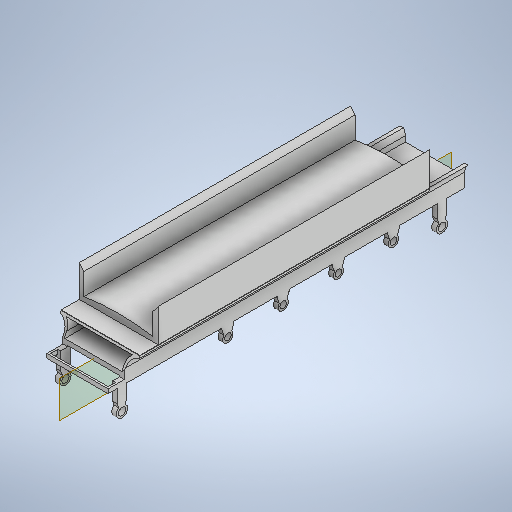
# Autodesk Inventor part: Wheel Holder of Train [Copy]
Saved by Autodesk Inventor 2025.1 (Build 291241020, 241B)
## iProperties
Created: 2022-11-30
Part Number: Wheel Holder of Train [Copy]
Material: Generic
Document SubType Name: Modeling
Designer: mc_vlongo24
Density: 1 g/cm^3
Appearance: Default
Author: mc_vlongo24
Autodesk Inventor part; units mm, degrees
ref_plane "YZ Plane" through (0, 0, 0) normal (1, 0, 0) x (0, 1, 0)
ref_plane "XZ Plane" through (0, 0, 0) normal (0, 1, 0) x (-1, 0, 0)
ref_plane "XY Plane" through (0, 0, 0) normal (0, 0, 1) x (1, 0, 0)
sketch "Sketch1" plane through (0, 0, 0) normal (0, 1, 0) x (-1, 0, 0)
  line L0 (25.5765, 3.2132) -> (-7.4435, 3.2132)
  line L1 (-7.4435, 3.2132) -> (-7.4435, -188.8108)
  line L2 (-7.4435, -188.8108) -> (25.5765, -188.8108)
  line L3 (25.5765, -188.8108) -> (25.5765, 3.2132)
  point P0 (0, 0)
  dimension "d0" = 33.02
  dimension "d1" = 192.024
  constraints: 8 end point, 2 parallel, 1 horizontal, 1 perpendicular
  measures "d0" distance of L2.end L1.end
  measures "d1" distance between parallel lines of L2 L0
extrude "Extrusion1" add sketch "Sketch1" against normal blind 23.8125
sketch "Sketch2" plane through (7.4435, 0, 3.2132) normal (1, 0, 0) x (0, 0, -1)
  line L0 (0, 0) -> (0, -23.8125) projected
  line L1 (192.024, 0) -> (192.024, -23.8125) projected
  line L2 (0, 0) -> (192.024, 0)
  line L3 (192.024, 0) -> (192.024, -20.9629)
  line L4 (192.024, -20.9629) -> (0, -20.9629)
  line L5 (0, -20.9629) -> (0, 0)
  point P0 (3.2132, 0)
  constraints: 8 end point, 2 parallel, 1 horizontal, 1 perpendicular, 1 point on line
extrude "Extrusion2" cut sketch "Sketch2" against normal blind 33.02
sketch "Sketch3" plane through (7.4435, -20.9629, 3.2132) normal (0, 1, 0) x (1, 0, 0)
  line L0 (-32.004, 1.016) -> (-1.016, 1.016)
  line L1 (-1.016, 1.016) -> (-1.016, 191.008)
  line L2 (-1.016, 191.008) -> (-32.004, 191.008)
  line L3 (-32.004, 191.008) -> (-32.004, 1.016)
  line L4 (-33.02, 192.024) -> (0, 192.024) projected
  line L5 (-33.02, 0) -> (-33.02, 192.024) projected
  line L6 (0, 192.024) -> (0, 0) projected
  line L7 (0, 0) -> (-33.02, 0) projected
  point P0 (-7.4435, 3.2132)
  dimension "d6" = 1.016
  dimension "d7" = 1.016
  dimension "d8" = 1.016
  dimension "d9" = 1.016
  constraints: 8 end point, 2 parallel, 1 horizontal, 1 perpendicular
  measures "d6" distance between parallel lines of L4 L2
  measures "d7" distance between parallel lines of L5 L3
  measures "d8" distance between parallel lines of L6 L1
  measures "d9" distance between parallel lines of L7 L0
extrude "Extrusion3" cut sketch "Sketch3" against normal blind 6.0325 contours L3 L2 L1 L0
sketch "Sketch4" plane through (7.4435, -23.8125, 3.2132) normal (1, 0, 0) x (0, 0, -1)
  line L0 (1.016, 2.8496) -> (191.008, 2.8496) projected
  line L1 (4.9428, 2.8496) -> (10.0228, 2.8496)
  line L2 (10.0228, 2.8496) -> (10.0228, -7.1834)
  line L3 (10.0228, -7.1834) -> (4.9428, -7.1834)
  line L4 (4.9428, -7.1834) -> (4.9428, 2.8496)
  circle A0 centre (7.4828, -12.0073) radius 2.032
  circle A1 centre (7.4828, -12.0073) radius 3.048
  line L5 (4.9428, -7.1834) -> (5.7788, -9.4802)
  line L6 (10.0228, -7.1834) -> (9.1869, -9.4802)
  circle A2 centre (64.4766, -5.6726) radius 1.7782
  circle A3 centre (94.2554, -5.6523) radius 1.7758
  circle A4 centre (123.9823, -5.6726) radius 1.766
  circle A5 centre (153.6687, -5.7132) radius 1.7937
  circle A6 centre (179.7884, -12.0369) radius 2.032
  circle A7 centre (179.7884, -12.0369) radius 3.048
  circle A8 centre (153.6687, -5.7132) radius 2.8097
  circle A9 centre (123.9823, -5.6726) radius 2.782
  circle A10 centre (94.2554, -5.6523) radius 2.7918
  circle A11 centre (64.4766, -5.6726) radius 2.7942
  line L7 (61.3016, 2.8496) -> (67.6516, 2.8496)
  line L8 (67.6516, 2.8496) -> (67.6516, -0.9604)
  line L9 (67.6516, -0.9604) -> (61.3016, -0.9604)
  line L10 (61.3016, -0.9604) -> (61.3016, 2.8496)
  line L11 (91.0804, 2.8496) -> (97.4304, 2.8496)
  line L12 (97.4304, 2.8496) -> (97.4304, -0.9604)
  line L13 (97.4304, -0.9604) -> (91.0804, -0.9604)
  line L14 (91.0804, -0.9604) -> (91.0804, 2.8496)
  line L15 (120.8073, 2.8496) -> (127.1573, 2.8496)
  line L16 (127.1573, 2.8496) -> (127.1573, -0.9604)
  line L17 (127.1573, -0.9604) -> (120.8073, -0.9604)
  line L18 (120.8073, -0.9604) -> (120.8073, 2.8496)
  line L19 (150.4937, 2.8496) -> (156.8437, 2.8496)
  line L20 (156.8437, 2.8496) -> (156.8437, -0.9604)
  line L21 (156.8437, -0.9604) -> (150.4937, -0.9604)
  line L22 (150.4937, -0.9604) -> (150.4937, 2.8496)
  line L23 (177.2484, 2.8496) -> (182.3284, 2.8496)
  line L24 (182.3284, 2.8496) -> (182.3284, -7.1834)
  line L25 (182.3284, -7.1834) -> (177.2484, -7.1834)
  line L26 (177.2484, -7.1834) -> (177.2484, 2.8496)
  line L27 (177.2484, -7.1834) -> (178.093, -9.5039)
  line L28 (182.3284, -7.1834) -> (181.4838, -9.5039)
  line L29 (61.3016, -0.9604) -> (62.3549, -3.8544)
  line L30 (67.6516, -0.9604) -> (66.5983, -3.8544)
  line L31 (91.0804, -0.9604) -> (92.1295, -3.8428)
  line L32 (97.4304, -0.9604) -> (96.3813, -3.8428)
  line L33 (120.8073, -0.9604) -> (121.8654, -3.8675)
  line L34 (127.1573, -0.9604) -> (126.0992, -3.8675)
  line L35 (150.4937, -0.9604) -> (151.5513, -3.8662)
  line L36 (156.8437, -0.9604) -> (155.7861, -3.8662)
  point P0 (3.2132, 23.8125)
  point P1 (10.0228, 2.8496)
  point P2 (127.1573, 2.8496)
  point P3 (156.8437, 2.8496)
  point P4 (182.3284, 2.8496)
  dimension "d12" = 1.016
  dimension "d13" = 1.016
  dimension "d14" = 1.016
  dimension "d15" = 1.016
  dimension "d16" = 1.016
  dimension "d17" = 1.016
  dimension "d18" = 5.08
  dimension "d19" = 6.35
  dimension "d21" = 2.54
  dimension "d22" = 4.064
  dimension "d23" = 4.064
  dimension "d24" = 5.08
  dimension "d25" = 2.54
  dimension "d26" = 10.033
  dimension "d27" = 70
  dimension "d28" = 70
  dimension "d29" = 70
  dimension "d30" = 70
  dimension "d31" = 10.033
  dimension "d32" = 3.175
  dimension "d33" = 6.35
  dimension "d34" = 6.35
  dimension "d35" = 6.35
  dimension "d36" = 3.175
  dimension "d37" = 3.175
  dimension "d38" = 3.175
  dimension "d39" = 3.81
  dimension "d40" = 3.81
  constraints: 72 end point, 18 parallel, 12 centre point, 12 point on circle, 8 point on line, 6 coincident, 6 horizontal, 6 perpendicular
  measures "d12" radial gap between concentric circles of A1 A0
  measures "d13" radial gap between concentric circles of A7 A6
  measures "d14" radial gap between concentric circles of A11 A2
  measures "d15" radial gap between concentric circles of A10 A3
  measures "d16" radial gap between concentric circles of A9 A4
  measures "d17" radial gap between concentric circles of A8 A5
  measures "d18" distance between parallel lines of L2 L4
  measures "d19" distance between parallel lines of L8 L10
  measures "d21" distance from line of A0.centre L4
  measures "d22" diameter of A0
  measures "d23" diameter of A6
  measures "d24" distance between parallel lines of L24 L26
  measures "d25" distance from line of A6.centre L26
  measures "d26" distance between parallel lines of L1 L3
  measures "d27" angle of L3 L5
  measures "d28" angle of L3 L6
  measures "d29" angle of L25 L27
  measures "d30" angle of L25 L28
  measures "d31" distance between parallel lines of L0 L25
  measures "d32" distance from line of A2.centre L10
  measures "d33" distance between parallel lines of L12 L14
  measures "d34" distance between parallel lines of L16 L18
  measures "d35" distance between parallel lines of L20 L22
  measures "d36" distance from line of L22 A5.centre
  measures "d37" distance from line of A4.centre L18
  measures "d38" distance from line of A3.centre L14
  measures "d39" distance between parallel lines of L7 L9
  measures "d40" distance between parallel lines of L0 L13
extrude "Extrusion4" add sketch "Sketch4" against normal blind 2.54
ref_plane "Work Plane1" through (-9.0665, -20.9629, -58.0884) normal (-1, 0, 0) x (0, 0, 1)
mirror "Mirror1" about plane through (-9.0665, -20.9629, -58.0884) normal (-1, 0, 0) of "Extrusion4"
sketch "Sketch5" plane through (7.4435, -20.9629, 3.2132) normal (0, 1, 0) x (1, 0, 0)
  line L0 (0, 0) -> (-33.02, 0) projected
  line L1 (0, 192.024) -> (0, 0) projected
  line L2 (-33.02, 0) -> (0, 0)
  line L3 (0, 0) -> (0, 192.024)
  line L4 (0, 192.024) -> (-33.02, 192.024)
  line L5 (-33.02, 192.024) -> (-33.02, 0)
  point P0 (-7.4435, 3.2132)
  constraints: 8 end point, 2 parallel, 1 horizontal, 1 perpendicular
extrude "Extrusion5" add sketch "Sketch5" along normal blind 2.54
sketch "Sketch8" plane through (-25.5765, -23.8125, 3.2132) normal (0, 0, 1) x (1, 0, 0)
  line L0 (0, 5.3896) -> (0, 0) projected
  line L1 (0, 5.3896) -> (0, 12.8895)
  line L2 (0, 12.8895) -> (-4.5789, 12.8895)
  line L3 (-4.5789, 12.8895) -> (-3.5629, 12.8895)
  line L4 (-3.5629, 12.8895) -> (-3.5629, 13.9055)
  line L5 (-3.5629, 13.9055) -> (-4.5789, 13.9055)
  line L6 (-4.5789, 13.9055) -> (-4.5789, 12.8895)
  line L7 (0, 5.3896) -> (33.02, 5.3896) projected
  line L8 (33.02, 5.3896) -> (33.02, 12.8895)
  line L9 (33.02, 12.8895) -> (37.846, 12.8895)
  line L10 (37.846, 12.8895) -> (36.83, 12.8895)
  line L11 (36.83, 12.8895) -> (36.83, 13.9055)
  line L12 (36.83, 13.9055) -> (37.846, 13.9055)
  line L13 (37.846, 13.9055) -> (37.846, 12.8895)
  line L14 (1.016, 5.3896) -> (1.016, 13.3975)
  line L15 (32.004, 5.3896) -> (32.004, 13.3975)
  line L16 (-3.5629, 13.9055) -> (1.016, 13.9055)
  line L17 (1.016, 13.9055) -> (1.016, 13.3975)
  line L18 (36.83, 13.9055) -> (32.004, 13.9055)
  line L19 (32.004, 13.3975) -> (32.004, 13.9055)
  point P0 (25.5765, 23.8125)
  point P1 (-4.0709, 12.8895)
  dimension "d45" = 4.826
  dimension "d47" = 1.016
  dimension "d48" = 1.016
  dimension "d50" = 1.016
  dimension "d51" = 1.016
  constraints: 36 end point, 7 point on line, 6 parallel, 4 horizontal, 4 vertical, 2 perpendicular, 1 midpoint
  measures "d45" distance of L8.end L9.end
  measures "d47" distance from line of point (-4.071, 12.889) L5
  measures "d48" distance between parallel lines of L10 L12
  measures "d50" distance between parallel lines of L8 L15
  measures "d51" distance between parallel lines of L14 L1
extrude "Extrusion6" add sketch "Sketch8" against normal blind 192.024
fillet "Fillet1" radius 5.588 4 edges at (7.4435, -10.923, -92.7988) (-25.5765, -10.923, -92.7988) (-24.5605, -9.907, -92.7988) (6.4275, -9.907, -92.7988)
sketch "Sketch9" plane through (-30.1554, -9.907, -188.8108) normal (-1, 0, 0) x (0, 0, 1)
  line L0 (192.024, -1.016) -> (0, -1.016) projected
  line L1 (192.024, 0) -> (0, 0) projected
  line L2 (192.024, -1.016) -> (192.024, 0)
  line L3 (192.024, 0) -> (0, 0)
  line L4 (0, 0) -> (0, -1.016)
  line L5 (0, -5.588) -> (0, 0) projected
  line L6 (0, -1.016) -> (0, 0) projected
  line L7 (0, -1.016) -> (192.024, -1.016)
  point P0 (188.8108, 9.907)
  dimension "d55" = 192.024
  dimension "d56" = 192.024
  constraints: 8 end point, 1 collinear, 1 horizontal, 1 point on line, 1 vertical
  measures "d55" distance of L1.start L1.end
  measures "d56" distance of L0.end L0.start
extrude "Extrusion7" add sketch "Sketch9" against normal blind 42.418
sketch "Sketch10" plane through (7.4435, -30.9959, -1.7296) normal (1, 0, 0) x (0, 0, -1)
  line L0 (-4.9428, 21.0889) -> (187.0812, 21.0889) projected
  line L1 (187.0812, 20.0729) -> (187.0812, 15.5009) projected
  line L2 (163.2797, 21.0889) -> (187.0812, 21.0889)
  line L3 (187.0812, 21.0889) -> (187.0812, 18.7027)
  line L4 (187.0812, 18.7027) -> (163.2797, 18.7027)
  line L5 (163.2797, 18.7027) -> (163.2797, 21.0889)
  point P0 (-1.7296, 30.9959)
  point P1 (187.0812, 20.0729)
  constraints: 8 end point, 2 parallel, 2 point on line, 1 horizontal, 1 perpendicular
extrude "Extrusion8" cut sketch "Sketch10" along normal mid plane 99.568
sketch "Sketch11" plane through (7.4435, -30.9959, -1.7296) normal (1, 0, 0) x (0, 0, -1)
  line L0 (-4.9428, 14.5767) -> (-4.9428, 7.1834) projected
  line L1 (-4.9428, 21.0889) -> (163.2797, 21.0889) projected
  line L2 (-4.9428, 9.4531) -> (3.7683, 9.4531)
  line L3 (3.7683, 9.4531) -> (3.7683, 21.0889)
  line L4 (3.7683, 21.0889) -> (-4.9428, 21.0889)
  line L5 (-4.9428, 21.0889) -> (-4.9428, 9.4531)
  line L6 (3.7683, 13.406) -> (7.3509, 21.0889)
  line L7 (7.3509, 21.0889) -> (-4.9428, 21.0889)
  point P0 (-1.7296, 30.9959)
  point P1 (-4.9428, 14.5767)
  dimension "d61" = 25
  constraints: 12 end point, 4 point on line, 2 parallel, 1 collinear, 1 horizontal, 1 perpendicular
  measures "d61" angle of L3 L6
extrude "Extrusion9" cut sketch "Sketch11" along normal mid plane 115.443
sketch "Sketch12" plane through (-30.1554, -9.907, -165.0093) normal (0, 1, 0) x (1, 0, 0)
  line L0 (0, -155.9288) -> (42.4249, -155.9288) projected
  line L1 (42.4249, -156.4026) -> (42.4249, 0) projected
  line L2 (0, -155.9288) -> (42.4249, -155.9288)
  line L3 (42.4249, -155.9288) -> (42.4249, -155.7812)
  line L4 (42.4249, -155.7812) -> (0, -155.7812)
  line L5 (0, -155.7812) -> (0, -155.9288)
  point P0 (30.1554, -165.0093)
  constraints: 8 end point, 2 parallel, 1 horizontal, 1 perpendicular, 1 point on line
extrude "Extrusion10" add sketch "Sketch12" along normal blind 0.254
sketch "Sketch13" plane through (-30.1554, -9.907, -9.0805) normal (0, 0, 1) x (1, 0, 0)
  line L0 (0, 0) -> (0, 0.254) projected
  line L1 (0, 0.254) -> (0, 17.3732)
  line L2 (0, 0.254) -> (42.4249, 0.254) projected
  line L3 (42.4249, 0.254) -> (42.4249, 17.3732)
  line L4 (42.4249, 17.3732) -> (42.4249, 18.1388)
  arc A0 (39.5323, 14.4073) -> (42.4249, 18.1388) centre (19.9053, 32.6091) ccw
  arc A1 (0, 17.3732) -> (2.3809, 14.413) centre (17.4913, 29.0041) ccw
  line L5 (2.3809, 14.413) -> (2.3809, 2.6954)
  line L6 (39.5323, 14.4073) -> (39.5323, 2.6798)
  arc A2 (39.5323, 2.6798) -> (2.3809, 2.6954) centre (20.9107, -106.7173) ccw
  point P0 (30.1554, 9.907)
  constraints: 10 end point, 6 point on circle, 3 centre point, 2 parallel, 2 vertical, 1 point on line
extrude "Extrusion11" add sketch "Sketch13" against normal blind 160.0835
sketch "Sketch14" plane through (-30.1554, -10.923, -165.0093) normal (-1, 0, 0) x (0, 0, 1)
  line L0 (155.9288, 1.016) -> (155.9288, 19.1548) projected
  line L1 (155.7812, 1.27) -> (-4.1547, 1.27) projected
  line L2 (155.9288, 19.1548) -> (146.118, 19.1548)
  line L3 (146.118, 19.1548) -> (146.118, 1.27)
  line L4 (146.118, 1.27) -> (155.9288, 1.27)
  line L5 (155.9288, 1.27) -> (155.9288, 19.1548)
  point P0 (165.0093, 10.923)
  constraints: 8 end point, 2 parallel, 1 horizontal, 1 perpendicular, 1 point on line
extrude "Extrusion12" cut sketch "Sketch14" against normal blind 160.0835
sketch "Sketch15" plane through (-30.1554, -9.653, -169.164) normal (-1, 0, 0) x (0, 0, 1)
  line L0 (159.9359, -0.254) -> (159.9359, 0) projected
  line L1 (159.9359, -0.254) -> (4.1547, -0.254) projected
  line L2 (159.9359, 0) -> (4.1547, 0)
  line L3 (4.1547, 0) -> (4.1547, -0.254)
  line L4 (4.1547, -0.254) -> (159.9359, -0.254)
  line L5 (159.9359, -0.254) -> (159.9359, 0)
  point P0 (169.164, 9.653)
  constraints: 8 end point, 2 parallel, 1 horizontal, 1 perpendicular
extrude "Extrusion13" add sketch "Sketch15" against normal blind 42.4256
sketch "Sketch16" plane through (-30.1554, -10.923, -165.0093) normal (-1, 0, 0) x (0, 0, 1)
  line L0 (0, 0) -> (0, -1.3702) projected
  line L1 (0, -0.1088) -> (-4.4347, -0.1088)
  line L2 (-4.4347, -0.1088) -> (-4.4347, 20.6785)
  line L3 (-4.4347, 20.6785) -> (0, 20.6785)
  line L4 (0, 20.6785) -> (0, -0.1088)
  point P0 (165.0093, 10.923)
  constraints: 8 end point, 2 parallel, 1 horizontal, 1 perpendicular, 1 point on line
extrude "Extrusion14" cut sketch "Sketch16" against normal blind 55.1256
body "Solid1"
